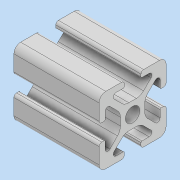
# Autodesk Inventor part: Extruson profile
Saved by Autodesk Inventor 2020 (Build 240168000, 168)
## iProperties
Created: 2020-04-09
Part Number: Extruson profile
Material: Generic
Document SubType Name: Modeling
Designer: Simon
Density: 1 g/cm^3
Appearance: Default
Author: Simon
Autodesk Inventor part; units mm, degrees
ref_plane "YZ Plane" through (0, 0, 0) normal (1, 0, 0) x (0, 1, 0)
ref_plane "XZ Plane" through (0, 0, 0) normal (0, 1, 0) x (-1, 0, 0)
ref_plane "XY Plane" through (0, 0, 0) normal (0, 0, 1) x (1, 0, 0)
sketch "Sketch1" plane through (0, 0, 0) normal (1, 0, 0) x (0, 1, 0)
  circle A0 centre (-3.2893, 9.9949) radius 2.1463
  line L0 (2.2183, 3.2343) -> (-0.0365, 5.4891)
  arc A1 (1.6256, 1.8034) -> (2.2183, 3.2343) centre (1.6256, 2.6416) ccw
  line L1 (-0.4826, 1.8034) -> (1.6256, 1.8034)
  arc A2 (-0.4826, 1.8034) -> (-0.7874, 1.4986) centre (-0.4826, 1.4986) ccw
  line L2 (-0.7874, 0.7874) -> (-0.7874, 1.4986)
  arc A3 (-0.7874, 0.7874) -> (0, 0) centre (0, 0.7874) ccw
  line L3 (4.699, 0) -> (0, 0)
  arc A4 (4.699, 0) -> (6.7056, 2.0066) centre (4.699, 2.0066) ccw
  line L4 (6.7056, 6.7056) -> (6.7056, 2.0066)
  arc A5 (6.7056, 6.7056) -> (5.9182, 7.493) centre (5.9182, 6.7056) ccw
  line L5 (5.207, 7.493) -> (5.9182, 7.493)
  arc A6 (5.207, 7.493) -> (4.9022, 7.1882) centre (5.207, 7.1882) ccw
  line L6 (4.9022, 5.08) -> (4.9022, 7.1882)
  arc A7 (3.4713, 4.4873) -> (4.9022, 5.08) centre (4.064, 5.08) ccw
  line L7 (1.2165, 6.7421) -> (3.4713, 4.4873)
  arc A8 (0.3386, 8.8615) -> (1.2165, 6.7421) centre (3.3358, 8.8615) ccw
  line L8 (0.3386, 11.1283) -> (0.3386, 8.8615)
  arc A9 (1.2165, 13.2477) -> (0.3386, 11.1283) centre (3.3358, 11.1283) ccw
  line L9 (3.4713, 15.5025) -> (1.2165, 13.2477)
  arc A10 (4.9022, 14.9098) -> (3.4713, 15.5025) centre (4.064, 14.9098) ccw
  line L10 (4.9022, 12.8016) -> (4.9022, 14.9098)
  arc A11 (4.9022, 12.8016) -> (5.207, 12.4968) centre (5.207, 12.8016) ccw
  line L11 (5.9182, 12.4968) -> (5.207, 12.4968)
  arc A12 (5.9182, 12.4968) -> (6.7056, 13.2842) centre (5.9182, 13.2842) ccw
  line L12 (6.7056, 17.9832) -> (6.7056, 13.2842)
  arc A13 (6.7056, 17.9832) -> (4.699, 19.9898) centre (4.699, 17.9832) ccw
  line L13 (0, 19.9898) -> (4.699, 19.9898)
  arc A14 (0, 19.9898) -> (-0.7874, 19.2024) centre (0, 19.2024) ccw
  line L14 (-0.7874, 18.4912) -> (-0.7874, 19.2024)
  arc A15 (-0.7874, 18.4912) -> (-0.4826, 18.1864) centre (-0.4826, 18.4912) ccw
  line L15 (1.6256, 18.1864) -> (-0.4826, 18.1864)
  arc A16 (2.2183, 16.7555) -> (1.6256, 18.1864) centre (1.6256, 17.3482) ccw
  line L16 (-0.0365, 14.5007) -> (2.2183, 16.7555)
  arc A17 (-2.1559, 13.6228) -> (-0.0365, 14.5007) centre (-2.1559, 16.62) ccw
  line L17 (-4.4227, 13.6228) -> (-2.1559, 13.6228)
  arc A18 (-6.5421, 14.5007) -> (-4.4227, 13.6228) centre (-4.4227, 16.62) ccw
  line L18 (-8.7969, 16.7555) -> (-6.5421, 14.5007)
  arc A19 (-8.2042, 18.1864) -> (-8.7969, 16.7555) centre (-8.2042, 17.3482) ccw
  line L19 (-6.096, 18.1864) -> (-8.2042, 18.1864)
  arc A20 (-6.096, 18.1864) -> (-5.7912, 18.4912) centre (-6.096, 18.4912) ccw
  line L20 (-5.7912, 19.2024) -> (-5.7912, 18.4912)
  arc A21 (-5.7912, 19.2024) -> (-6.5786, 19.9898) centre (-6.5786, 19.2024) ccw
  line L21 (-11.2776, 19.9898) -> (-6.5786, 19.9898)
  arc A22 (-11.2776, 19.9898) -> (-13.2842, 17.9832) centre (-11.2776, 17.9832) ccw
  line L22 (-13.2842, 13.2842) -> (-13.2842, 17.9832)
  arc A23 (-13.2842, 13.2842) -> (-12.4968, 12.4968) centre (-12.4968, 13.2842) ccw
  line L23 (-11.7856, 12.4968) -> (-12.4968, 12.4968)
  arc A24 (-11.7856, 12.4968) -> (-11.4808, 12.8016) centre (-11.7856, 12.8016) ccw
  line L24 (-11.4808, 14.9098) -> (-11.4808, 12.8016)
  arc A25 (-10.0499, 15.5025) -> (-11.4808, 14.9098) centre (-10.6426, 14.9098) ccw
  line L25 (-7.7951, 13.2477) -> (-10.0499, 15.5025)
  arc A26 (-6.9172, 11.1283) -> (-7.7951, 13.2477) centre (-9.9144, 11.1283) ccw
  line L26 (-6.9172, 8.8615) -> (-6.9172, 11.1283)
  arc A27 (-7.7951, 6.7421) -> (-6.9172, 8.8615) centre (-9.9144, 8.8615) ccw
  line L27 (-10.0499, 4.4873) -> (-7.7951, 6.7421)
  arc A28 (-11.4808, 5.08) -> (-10.0499, 4.4873) centre (-10.6426, 5.08) ccw
  line L28 (-11.4808, 7.1882) -> (-11.4808, 5.08)
  arc A29 (-11.4808, 7.1882) -> (-11.7856, 7.493) centre (-11.7856, 7.1882) ccw
  line L29 (-12.4968, 7.493) -> (-11.7856, 7.493)
  arc A30 (-12.4968, 7.493) -> (-13.2842, 6.7056) centre (-12.4968, 6.7056) ccw
  line L30 (-13.2842, 2.0066) -> (-13.2842, 6.7056)
  arc A31 (-13.2842, 2.0066) -> (-11.2776, 0) centre (-11.2776, 2.0066) ccw
  line L31 (-6.5786, 0) -> (-11.2776, 0)
  arc A32 (-6.5786, 0) -> (-5.7912, 0.7874) centre (-6.5786, 0.7874) ccw
  line L32 (-5.7912, 1.4986) -> (-5.7912, 0.7874)
  arc A33 (-5.7912, 1.4986) -> (-6.096, 1.8034) centre (-6.096, 1.4986) ccw
  line L33 (-8.2042, 1.8034) -> (-6.096, 1.8034)
  arc A34 (-8.7969, 3.2343) -> (-8.2042, 1.8034) centre (-8.2042, 2.6416) ccw
  line L34 (-6.5421, 5.4891) -> (-8.7969, 3.2343)
  arc A35 (-4.4227, 6.367) -> (-6.5421, 5.4891) centre (-4.4227, 3.3698) ccw
  line L35 (-2.1559, 6.367) -> (-4.4227, 6.367)
  arc A36 (-0.0365, 5.4891) -> (-2.1559, 6.367) centre (-2.1559, 3.3698) ccw
  constraints: 72 end point, 72 point on circle, 37 centre point, 14 horizontal, 14 vertical, 156 other
extrude "Extrusion1" add sketch "Sketch1" along normal blind 25.4
body "Solid1"
